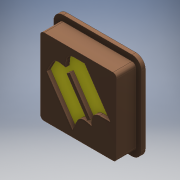
# Autodesk Inventor part: button4
Saved by Autodesk Inventor 2016 (Build 200138000, 138)
## iProperties
Created: 2017-11-06
Part Number: button4
Material: Bronze, Soft Tin
Document SubType Name: Modeling
Designer: Davide
Density: 8.874 g/cm^3
Appearance: Bronze - Satin
Author: Davide
Autodesk Inventor part; units mm, degrees
ref_plane "YZ Plane" through (0, 0, 0) normal (1, 0, 0) x (0, 1, 0)
ref_plane "XZ Plane" through (0, 0, 0) normal (0, 1, 0) x (-1, 0, 0)
ref_plane "XY Plane" through (0, 0, 0) normal (0, 0, 1) x (1, 0, 0)
sketch "Sketch1" plane through (0, 0, 0) normal (0, 1, 0) x (-1, 0, 0)
  line L0 (9, -10) -> (-9, -10)
  line L1 (-10, -9) -> (-10, 9)
  line L2 (-9, 10) -> (9, 10)
  line L3 (10, 9) -> (10, -9)
  line L4 (10, 10) -> (-10, -10) construction
  line L5 (10, -10) -> (-10, 10) construction
  arc A0 (10, 9) -> (9, 10) centre (9, 9) ccw
  arc A1 (9, -10) -> (10, -9) centre (9, -9) ccw
  arc A2 (-10, -9) -> (-9, -10) centre (-9, -9) ccw
  arc A3 (-9, 10) -> (-10, 9) centre (-9, 9) ccw
  point P0 (0, 0)
  point P1 (0, 0)
  dimension "d7" = 20
  dimension "d9" = 20
  dimension "d10" = 1
  constraints: 12 end point, 8 point on circle, 8 point on line, 8 tangent, 4 centre point, 3 equal radius, 2 parallel, 1 coincident, 1 horizontal, 1 midpoint, 1 perpendicular
  measures "d7" distance of L5.start L4.end
  measures "d9" distance of L4.end L5.end
  measures "d10" radius of A0
extrude "Extrusion1" add sketch "Sketch1" along normal blind 5
sketch "Sketch2" plane through (0, 5, 0) normal (0, 1, 0) x (1, 0, 0)
  line L0 (-10, 9) -> (-10, -9) projected
  arc A0 (-10, -9) -> (-9, -10) centre (-9, -9) ccw projected
  line L1 (-9, -10) -> (9, -10) projected
  arc A1 (9, -10) -> (10, -9) centre (9, -9) ccw projected
  line L2 (10, -9) -> (10, 9) projected
  arc A2 (10, 9) -> (9, 10) centre (9, 9) ccw projected
  line L3 (9, 10) -> (-9, 10) projected
  arc A3 (-9, 10) -> (-10, 9) centre (-9, 9) ccw projected
  line L4 (9, -11.5) -> (-9, -11.5)
  arc A4 (-11.5, -9) -> (-9, -11.5) centre (-9, -9) ccw
  line L5 (-11.5, -9) -> (-11.5, 9)
  arc A5 (-9, 11.5) -> (-11.5, 9) centre (-9, 9) ccw
  line L6 (-9, 11.5) -> (9, 11.5)
  arc A6 (11.5, 9) -> (9, 11.5) centre (9, 9) ccw
  line L7 (11.5, 9) -> (11.5, -9)
  arc A7 (9, -11.5) -> (11.5, -9) centre (9, -9) ccw
  circle A8 centre (0, 0) radius 2.75
  dimension "d16" = 1.5
  dimension "d19" = 5.5
  constraints: 8 end point, 8 point on circle, 5 centre point, 1 coincident, 7 other
  measures "d16" distance between parallel lines of L1 L4
  measures "d19" diameter of A8
extrude "Extrusion3" add sketch "Sketch2" along normal blind 1 contours A3 L3 A2 L2 A1 L1 A0 L0 | L4 A4 L5 A5 L6 A6 L7 A7
sketch "Sketch3" plane through (0, 0, 0) normal (0, -1, 0) x (1, 0, 0)
  line L0 (-8.3335, 1.5979) -> (-1.5979, -8.3335)
  line L1 (-1.5979, -8.3335) -> (-0.3669, -5.7051)
  line L2 (1.9204, -4.6109) -> (3.3678, -4.9657)
  line L3 (3.3678, -4.9657) -> (3.4632, -3.4705)
  line L4 (5.4592, -1.5979) -> (8.3335, -1.5979)
  line L5 (8.3335, -1.5979) -> (1.5979, 8.3335)
  line L6 (1.5979, 8.3335) -> (-1.2764, 8.3335)
  line L7 (-3.2724, 6.4609) -> (-3.3678, 4.9657)
  line L8 (-3.3678, 4.9657) -> (-4.8403, 5.2316)
  line L9 (-6.9654, 4.1955) -> (-8.3335, 1.5979)
  line L10 (-3.3678, 4.9657) -> (3.3678, -4.9657) construction
  arc A0 (-4.8403, 5.2316) -> (-6.9654, 4.1955) centre (-5.1958, 3.2635) ccw
  arc A1 (-1.2764, 8.3335) -> (-3.2724, 6.4609) centre (-1.2764, 6.3335) ccw
  arc A2 (5.4592, -1.5979) -> (3.4632, -3.4705) centre (5.4592, -3.5979) ccw
  arc A3 (1.9204, -4.6109) -> (-0.3669, -5.7051) centre (1.4443, -6.5534) ccw
  line L11 (-4.9657, -3.3678) -> (0, 0) construction
  line L12 (0, 0) -> (4.9657, 3.3678) construction
  line L13 (-2.6449, 7.792) -> (4.0907, -2.1393) construction
  line L14 (-2.7456, 0.156) -> (0.8707, 2.6085) construction
  circle A4 centre (0, 0) radius 2.75 construction
  line L15 (-6.0723, 5.0611) -> (0.5812, -4.7492) construction
  line L16 (-3.0915, 3.7031) -> (2.297, -4.242)
  line L17 (2.297, -4.242) -> (3.0915, -3.7031)
  line L18 (3.0915, -3.7031) -> (-2.297, 4.242)
  line L19 (-2.297, 4.242) -> (-3.0915, 3.7031)
  point P0 (-0.9375, 1.3822)
  point P1 (-2.6942, 3.9725)
  point P2 (2.6942, -3.9725)
  point P3 (-0.3973, -0.2694)
  dimension "d77" = 2
  dimension "d78" = 12
  dimension "d79" = 12
  dimension "d80" = 12
  dimension "d81" = 6
  dimension "d82" = 6
  dimension "d85" = 9.6
  dimension "d86" = 0.96
  constraints: 40 end point, 12 point on circle, 8 midpoint, 8 tangent, 6 parallel, 5 point on line, 4 centre point, 4 perpendicular, 3 equal radius, 1 coincident, 1 collinear, 1 horizontal, 2 other
  measures "d77" radius of A0
  measures "d78" distance of L0.start L0.end
  measures "d79" distance of L7.end L2.end
  measures "d80" distance of L4.end L5.end
  measures "d81" distance of L11.start L11.end
  measures "d82" distance of L11.end L12.end
  measures "d85" distance of L16.start L16.end
  measures "d86" distance between parallel lines of L18 L16
extrude "Extrusion7" cut sketch "Sketch3" against normal blind 1
extrude "Extrusion8" cut sketch "Sketch2" against normal blind 2 contours A8
equation "\"d7\" = button_side"
equation "\"d9\" = d7"
equation "\"d78\" = d79"
equation "\"d79\" = 0.6 * button_side"
equation "\"d80\" = d79"
equation "\"d81\" = d82"
equation "\"d82\" = 0.5 * d79"
equation "\"d85\" = 0.8 * d80"
equation "\"d86\" = 0.1 * d85"
equation "\"d0\" = 122"
equation "\"d1\" = 77"
equation "\"d4\" = 19"
equation "\"d5\" = 1"
equation "\"d8\" = 25"
equation "\"d13\" = 1.5"
equation "\"d14\" = 0"
equation "\"d15\" = 2"
equation "\"d30\" = 3.1"
equation "\"d31\" = 3"
equation "\"d33\" = 3"
equation "\"d34\" = 2"
equation "\"d36\" = 3"
equation "\"d38\" = 90deg"
equation "\"d39\" = 8"
equation "\"d40\" = 118deg"
equation "\"d44\" = 0"
equation "\"d45\" = 1.2"
equation "\"d46\" = 2"
equation "\"d47\" = 0"
equation "\"d50\" = 25"
equation "\"button_side\" = 20"
equation "\"d3\" = 1.01 * button_side"
equation "\"d2\" = d3"
body "Solid1"
